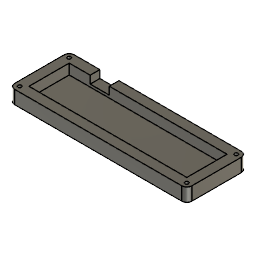
Celeste Hackpad Base (Autodesk Fusion 360 design; units mm, degrees)
part number: 2025-12-01-20-37-59-941
Autodesk Fusion 360 part; units mm, degrees
sketch "Sketch1" plane through (0, 0, 0) normal (0, 0, 1) x (1, 0, 0)
  line L0 (0, 0) -> (153.4, 0)
  line L1 (153.4, 0) -> (153.4, -39.1)
  line L2 (153.4, -39.1) -> (0, -39.1)
  line L3 (0, -39.1) -> (0, 0)
  line L4 (-9.5, 9.5) -> (162.9, 9.5)
  line L5 (162.9, 9.5) -> (162.9, -48.6)
  line L6 (162.9, -48.6) -> (-9.5, -48.6)
  line L7 (-9.5, -48.6) -> (-9.5, 9.5)
  circle A0 centre (-4.5, 4.5) radius 1.7
  circle A1 centre (-4.5, -43.6) radius 1.7
  circle A2 centre (-4.5, -43.6) radius 3
  circle A3 centre (-4.5, 4.5) radius 3
  circle A4 centre (157.9, 4.5) radius 1.7
  circle A5 centre (157.9, 4.5) radius 3
  circle A6 centre (157.9, -43.6) radius 1.7
  circle A7 centre (157.9, -43.6) radius 3
  dimension "d1" = 153.4
  dimension "d2" = 39.1
  dimension "d3" = 172.4
  dimension "d4" = 58.1
  dimension "d5" = 9.5
  dimension "d6" = 9.5
  dimension "d7" = 3.4
  dimension "d8" = 5
  dimension "d9" = 5
  dimension "d10" = 3.4
  dimension "d11" = 5
  dimension "d12" = 5
  dimension "d13" = 6
  dimension "d14" = 6
  dimension "d15" = 3.4
  dimension "d16" = 5
  dimension "d17" = 5
  dimension "d18" = 6
  dimension "d19" = 3.4
  dimension "d20" = 5
  dimension "d21" = 5
  dimension "d22" = 6
  constraint horizontal L0
  constraint vertical L1
  constraint horizontal L2
  constraint vertical L3
  constraint coincident L0.start L3.end
  constraint horizontal L4
  constraint vertical L5
  constraint horizontal L6
  constraint vertical L7
  constraint concentric A1 A2
  constraint concentric A0 A3
  constraint concentric A4 A5
  constraint concentric A6 A7
  measures "d1" distance of L0.start L0.end
  measures "d2" distance of L0.start L2.end
  measures "d3" distance of L4.start L4.end
  measures "d4" distance of L4.start L6.end
  measures "d5" distance of L0 L4
  measures "d6" distance of L3 L7
  measures "d7" diameter of A0
  measures "d8" distance of L4 A0.centre
  measures "d9" distance of L7 A0.centre
  measures "d10" diameter of A1
  measures "d11" distance of L6 A1.centre
  measures "d12" distance of L7 A1.centre
  measures "d13" diameter of A2
  measures "d14" diameter of A3
  measures "d15" diameter of A4
  measures "d16" distance of L5 A4.centre
  measures "d17" distance of L4 A4.centre
  measures "d18" diameter of A5
  measures "d19" diameter of A6
  measures "d20" distance of L6 A6.centre
  measures "d21" distance of L5 A6.centre
  measures "d22" diameter of A7
extrude "Extrude1" add sketch "Sketch1" along normal blind 9.9 from surface at 3.1 contours A2 | A3 | A5 | A7 makes body 1 at (-1.5037, 4.3505, 9.7) makes body 2 at (160.1981, 6.4284, 9.7) makes body 3 at (-1.5037, -43.7495, 9.7) makes body 4 at (159.9947, -41.4524, 9.7)
extrude "Extrude2" add sketch "Sketch1" along normal blind 13 contours L4 L5 L6 L7 bodies 1 2 3 4
extrude "Extrude3" add sketch "Sketch1" along normal blind 3 contours L0 L1 L2 L3 bodies 1
sketch "Sketch2" plane through (0, 0, 13) normal (0, 0, 1) x (-1, 0, 0)
  circle A0 centre (4.5, -4.5) radius 1.7
  circle A1 centre (-157.9, 43.6) radius 1.7
  line L0 (-153.4, 39.1) -> (0, 39.1)
  line L1 (0, 39.1) -> (0, 0)
  line L2 (0, 0) -> (-153.4, 0)
  line L3 (-153.4, 0) -> (-153.4, 39.1)
  line L4 (9.5, 48.6) -> (-162.9, 48.6)
  line L5 (-162.9, 48.6) -> (-162.9, -9.5)
  line L6 (-162.9, -9.5) -> (9.5, -9.5)
  line L7 (9.5, -9.5) -> (9.5, 48.6)
  circle A2 centre (-157.9, -4.5) radius 1.7
  circle A3 centre (4.5, 43.6) radius 1.7
  line L8 (-20.386, -9.5) -> (-38.886, -9.5)
  line L9 (-38.886, -9.5) -> (-38.886, 0)
  line L10 (-38.886, 0) -> (-20.386, 0)
  line L11 (-20.386, 0) -> (-20.386, -9.5)
  dimension "d30" = 18.5
  dimension "d31" = 29.886
  constraint horizontal L8
  constraint vertical L9
  constraint horizontal L10
  constraint vertical L11
  constraint coincident L6 L8.start
  measures "d30" distance of L8.start L8.end
  measures "d31" distance of L7 L11
extrude "Extrude4" cut sketch "Sketch2" against normal blind 7.5 contours L2 L6 L8 L9 L10 L11 bodies 1
fillet "Fillet1" radius 5 4 edges at (-9.5, -48.6, 6.5) (-9.5, 9.5, 6.5) (162.9, 9.5, 6.5) (162.9, -48.6, 6.5) on bodies 1
